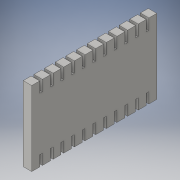
# Autodesk Inventor part: frame_side
Saved by Autodesk Inventor 2016 (Build 200138000, 138)
## iProperties
Created: 2017-09-21
Part Number: frame_side
Material: Generic
Document SubType Name: Modeling
Designer: Student
Density: 1 g/cm^3
Appearance: Default
Author: Student
Autodesk Inventor part; units mm, degrees
ref_plane "YZ Plane" through (0, 0, 0) normal (1, 0, 0) x (0, 1, 0)
ref_plane "XZ Plane" through (0, 0, 0) normal (0, 1, 0) x (-1, 0, 0)
ref_plane "XY Plane" through (0, 0, 0) normal (0, 0, 1) x (1, 0, 0)
sketch "Sketch1" plane through (0, 0, 0) normal (1, 0, 0) x (0, 1, 0)
  line L0 (0, 0) -> (25.4, 0)
  line L1 (0, 0) -> (-5.08, 0)
  line L2 (-5.08, 0) -> (-5.08, -3.81)
  line L3 (-5.08, -3.81) -> (0, -3.81)
  line L4 (25.4, 0) -> (30.48, 0)
  line L5 (30.48, 0) -> (30.48, -3.81)
  line L6 (30.48, -3.81) -> (25.4, -3.81)
  line L7 (25.4, -5.08) -> (30.48, -5.08)
  line L8 (30.48, -5.08) -> (30.48, -8.89)
  line L9 (30.48, -8.89) -> (25.4, -8.89)
  line L10 (25.4, -10.16) -> (30.48, -10.16)
  line L11 (30.48, -10.16) -> (30.48, -13.97)
  line L12 (30.48, -13.97) -> (25.4, -13.97)
  line L13 (25.4, -15.24) -> (30.48, -15.24)
  line L14 (30.48, -15.24) -> (30.48, -19.05)
  line L15 (30.48, -19.05) -> (25.4, -19.05)
  line L16 (25.4, -20.32) -> (30.48, -20.32)
  line L17 (30.48, -20.32) -> (30.48, -24.13)
  line L18 (30.48, -24.13) -> (25.4, -24.13)
  line L19 (25.4, -25.4) -> (30.48, -25.4)
  line L20 (30.48, -25.4) -> (30.48, -29.21)
  line L21 (30.48, -29.21) -> (25.4, -29.21)
  line L22 (25.4, -30.48) -> (30.48, -30.48)
  line L23 (30.48, -30.48) -> (30.48, -34.29)
  line L24 (30.48, -34.29) -> (25.4, -34.29)
  line L25 (25.4, -35.56) -> (30.48, -35.56)
  line L26 (30.48, -35.56) -> (30.48, -39.37)
  line L27 (30.48, -39.37) -> (25.4, -39.37)
  line L28 (25.4, -40.64) -> (30.48, -40.64)
  line L29 (30.48, -40.64) -> (30.48, -44.45)
  line L30 (30.48, -44.45) -> (25.4, -44.45)
  line L31 (25.4, -45.72) -> (30.48, -45.72)
  line L32 (30.48, -45.72) -> (30.48, -49.53)
  line L33 (30.48, -49.53) -> (25.4, -49.53)
  line L34 (25.4, -50.8) -> (30.48, -50.8)
  line L35 (30.48, -50.8) -> (30.48, -54.61)
  line L36 (30.48, -54.61) -> (25.4, -54.61)
  line L37 (25.4, -55.88) -> (30.48, -55.88)
  line L38 (30.48, -55.88) -> (30.48, -59.69)
  line L39 (25.4, -5.08) -> (25.4, -3.81)
  line L40 (25.4, -10.16) -> (25.4, -8.89)
  line L41 (25.4, -15.24) -> (25.4, -13.97)
  line L42 (25.4, -20.32) -> (25.4, -19.05)
  line L43 (25.4, -25.4) -> (25.4, -24.13)
  line L44 (25.4, -30.48) -> (25.4, -29.21)
  line L45 (25.4, -35.56) -> (25.4, -34.29)
  line L46 (25.4, -40.64) -> (25.4, -39.37)
  line L47 (25.4, -45.72) -> (25.4, -44.45)
  line L48 (25.4, -55.88) -> (25.4, -54.61)
  line L49 (25.4, -50.8) -> (25.4, -49.53)
  line L50 (0, -5.08) -> (0, -3.81)
  line L51 (0, -10.16) -> (0, -8.89)
  line L52 (0, -15.24) -> (0, -13.97)
  line L53 (0, -20.32) -> (0, -19.05)
  line L54 (0, -25.4) -> (0, -24.13)
  line L55 (0, -30.48) -> (0, -29.21)
  line L56 (0, -35.56) -> (0, -34.29)
  line L57 (0, -40.64) -> (0, -39.37)
  line L58 (0, -45.72) -> (0, -44.45)
  line L59 (0, -55.88) -> (0, -54.61)
  line L60 (0, -50.8) -> (0, -49.53)
  line L61 (30.48, -59.69) -> (-5.08, -59.69)
  line L62 (12.7, -59.69) -> (12.7, -46.4119) construction
  line L63 (-5.08, -5.08) -> (-5.08, -8.89)
  line L64 (-5.08, -8.89) -> (0, -8.89)
  line L65 (0, -20.32) -> (-5.08, -20.32)
  line L66 (-5.08, -24.13) -> (0, -24.13)
  line L67 (-5.08, -20.32) -> (-5.08, -24.13)
  line L68 (0, -25.4) -> (-5.08, -25.4)
  line L69 (-5.08, -25.4) -> (-5.08, -29.21)
  line L70 (0, -5.08) -> (-5.08, -5.08)
  line L71 (-5.08, -3.81) -> (0, -3.81)
  line L72 (0, 0) -> (-5.08, 0)
  line L73 (-5.08, 0) -> (-5.08, -3.81)
  line L74 (-5.08, -29.21) -> (0, -29.21)
  line L75 (0, -35.56) -> (-5.08, -35.56)
  line L76 (-5.08, -34.29) -> (0, -34.29)
  line L77 (0, -30.48) -> (-5.08, -30.48)
  line L78 (-5.08, -30.48) -> (-5.08, -34.29)
  line L79 (-5.08, -39.37) -> (0, -39.37)
  line L80 (-5.08, -35.56) -> (-5.08, -39.37)
  line L81 (0, -40.64) -> (-5.08, -40.64)
  line L82 (-5.08, -44.45) -> (0, -44.45)
  line L83 (0, -45.72) -> (-5.08, -45.72)
  line L84 (-5.08, -45.72) -> (-5.08, -49.53)
  line L85 (-5.08, -40.64) -> (-5.08, -44.45)
  line L86 (-5.08, -49.53) -> (0, -49.53)
  line L87 (0, -50.8) -> (-5.08, -50.8)
  line L88 (-5.08, -50.8) -> (-5.08, -54.61)
  line L89 (-5.08, -54.61) -> (0, -54.61)
  line L90 (0, -55.88) -> (-5.08, -55.88)
  line L91 (-5.08, -55.88) -> (-5.08, -59.69)
  line L92 (-5.08, -19.05) -> (0, -19.05)
  line L93 (0, -15.24) -> (-5.08, -15.24)
  line L94 (-5.08, -15.24) -> (-5.08, -19.05)
  line L95 (-5.08, -13.97) -> (0, -13.97)
  line L96 (0, -10.16) -> (-5.08, -10.16)
  line L97 (-5.08, -10.16) -> (-5.08, -13.97)
  line L98 (0, -5.08) -> (0, -3.81)
  line L99 (0, -10.16) -> (0, -8.89)
  line L100 (0, -15.24) -> (0, -13.97)
  line L101 (0, -20.32) -> (0, -19.05)
  line L102 (0, -25.4) -> (0, -24.13)
  line L103 (0, -30.48) -> (0, -29.21)
  line L104 (0, -35.56) -> (0, -34.29)
  line L105 (0, -40.64) -> (0, -39.37)
  line L106 (0, -45.72) -> (0, -44.45)
  line L107 (0, -55.88) -> (0, -54.61)
  line L108 (0, -50.8) -> (0, -49.53)
  dimension "d13" = 5.08
  constraints: 218 end point, 21 symmetric about line, 3 horizontal, 1 midpoint, 1 parallel, 1 perpendicular, 1 vertical
  measures "d13" distance of L0.start L50.start
extrude "Extrusion1" add sketch "Sketch1" along normal blind 4.064
body "Solid1"
